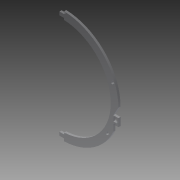
# Autodesk Inventor part: BottomHoop_v1
Saved by Autodesk Inventor 2013 (Build 170138000, 138)
## iProperties
Created: 2013-01-17
Part Number: BottomHoop_v1
Material: Polycarbonate, Clear
Document SubType Name: Modeling
Designer: motoennies
Density: 1.2 g/cm^3
Mass: 83.6781 g
Surface Area: 294.544 cm^2
Volume: 69.7318 cm^3
Author: motoennies
Autodesk Inventor part; units mm, degrees
ref_plane "YZ Plane" through (0, 0, 0) normal (1, 0, 0) x (0, 1, 0)
ref_plane "XZ Plane" through (0, 0, 0) normal (0, 1, 0) x (-1, 0, 0)
ref_plane "XY Plane" through (0, 0, 0) normal (0, 0, 1) x (1, 0, 0)
sketch "Sketch1" plane through (0, 0, 0) normal (0, 0, 1) x (1, 0, 0)
  arc A0 (6.35, -145.9119) -> (0, 146.05) centre (0, 0) ccw
  line L0 (0, 0) -> (0, 323.4187) construction
  line L1 (0, 0) -> (0, -168.91) construction
  line L2 (6.35, -168.7906) -> (6.35, -145.9119)
  line L3 (6.35, 145.9119) -> (6.35, 168.7906)
  line L4 (0, -146.05) -> (0, -151.13)
  line L5 (0, -151.13) -> (6.35, -151.13)
  line L6 (6.35, -151.13) -> (-7.62, -151.13)
  line L7 (-7.62, -151.13) -> (-7.62, -161.29)
  line L8 (-7.62, -161.29) -> (6.35, -161.29)
  line L9 (0, 146.05) -> (0, 151.13)
  line L10 (0, 151.13) -> (6.35, 151.13)
  line L11 (6.35, 151.13) -> (-7.62, 151.13)
  line L12 (-7.62, 151.13) -> (-7.62, 161.29)
  line L13 (-7.62, 161.29) -> (6.35, 161.29)
  line L14 (168.91, 0) -> (168.91, -50.8)
  line L15 (168.91, -50.8) -> (161.0899, -50.8)
  arc A1 (168.91, 0) -> (6.35, 168.7906) centre (0, 0) ccw
  arc A2 (6.35, -168.7906) -> (161.0899, -50.8) centre (0, 0) ccw
  dimension "d0" = 292.1
  dimension "d7" = 6.35
  dimension "d8" = 6.35
  dimension "d9" = 5.08
  dimension "d10" = 13.97
  dimension "d11" = 10.16
  dimension "d12" = 5.08
  dimension "d13" = 13.97
  dimension "d14" = 10.16
  dimension "d15" = 50.8
  dimension "d16" = 5.2181
  constraints: 32 end point, 9 point on line, 8 perpendicular, 7 point on circle, 3 centre point, 3 collinear, 2 coincident, 1 tangent, 1 vertical, 2 other
  measures "d0" diameter of A0
  measures "d7" distance between parallel lines of L2 L1
  measures "d8" distance between parallel lines of L0 L3
  measures "d9" distance of L4.start L4.end
  measures "d10" distance of L5.end L6.end
  measures "d11" distance of L6.end L7.end
  measures "d12" distance of L9.start L9.end
  measures "d13" distance of L10.end L11.end
  measures "d14" distance of L11.end L12.end
  measures "d15" distance of L14.start L14.end
  measures "d16" distance from line of L5 L2.end
extrude "Extrusion2" add sketch "Sketch1" along normal blind 6.35 contours A0 L3 A1 L14 L15 A2 L2 | L2 L8 L7 L6 L5 | L10 L11 L12 L13 L3
sketch "Sketch2" plane through (0, 0, 6.35) normal (0, 0, 1) x (1, 0, 0)
  line L0 (168.91, -50.8) -> (168.91, 0) projected
  line L1 (168.91, -50.8) -> (168.91, -43.2308)
  line L2 (168.91, -43.2308) -> (163.83, -43.2308)
  line L3 (163.83, -43.2308) -> (153.67, -43.2308)
  line L4 (153.67, -43.2308) -> (153.67, -33.7058)
  line L5 (153.67, -33.7058) -> (163.83, -33.7058)
  line L6 (163.83, -33.7058) -> (163.83, -43.2308)
  arc A0 (6.35, -168.7906) -> (161.0899, -50.8) centre (0, 0) ccw projected
  line L7 (161.0899, -50.8) -> (168.91, -50.8) projected
  arc A1 (168.91, 0) -> (6.35, 168.7906) centre (0, 0) ccw projected
  line L8 (168.91, -50.8) -> (153.67, -50.8)
  line L9 (153.67, -50.8) -> (153.67, -70.115)
  line L10 (153.67, -70.115) -> (168.91, -70.115)
  line L11 (168.91, -70.115) -> (168.91, -50.8)
  line L12 (168.91, -50.8) -> (168.91, -27.3558) construction
  line L13 (168.91, -27.3558) -> (153.67, -27.3558)
  line L14 (153.67, -27.3558) -> (168.91, 0)
  line L15 (168.91, -27.3558) -> (168.91, 0)
  dimension "d21" = 7.5692
  dimension "d22" = 5.08
  dimension "d23" = 10.16
  dimension "d24" = 9.525
  dimension "d27" = 15.24
  dimension "d28" = 23.4442
  dimension "d29" = 15.24
  constraints: 28 end point, 7 perpendicular, 3 point on line, 2 collinear, 1 parallel, 1 point on circle, 1 tangent
  measures "d21" distance of L0.start L1.end
  measures "d22" distance of L1.end L2.end
  measures "d23" distance of L2.end L3.end
  measures "d24" distance of L3.end L4.end
  measures "d27" distance of L0.start L8.end
  measures "d28" distance of L0.start L12.end
  measures "d29" distance of L12.end L13.end
extrude "Extrusion4" cut sketch "Sketch2" against normal blind 25.4 contours L13 L14 L0 | L3 L4 L5 L6 | L9 L8 A0
sketch "Sketch4" plane through (0, 0, 6.35) normal (0, 0, 1) x (1, 0, 0)
  circle A0 centre (149.4633, 54.61) radius 3.3782 projected
  circle A1 centre (134.268, -85.09) radius 3.3782 projected
extrude "Extrusion6" cut sketch "Sketch4" against normal blind 25.4
body "Solid2"
